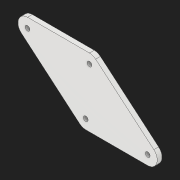
# Autodesk Inventor part: HA014
Saved by Autodesk Inventor 2017 SP1 (Build 210196100, 196)
## iProperties
Created: 2018-02-28
Part Number: HA014
Material: ABS Plastic
Document SubType Name: Modeling
Designer: Zach
Density: 1.06 g/cm^3
Appearance: CR White
Author: Zach
Autodesk Inventor part; units mm, degrees
ref_plane "YZ Plane" through (0, 0, 0) normal (1, 0, 0) x (0, 1, 0)
ref_plane "XZ Plane" through (0, 0, 0) normal (0, 1, 0) x (-1, 0, 0)
ref_plane "XY Plane" through (0, 0, 0) normal (0, 0, 1) x (1, 0, 0)
sketch "Sketch1" plane through (0, 0, 0) normal (0, 0, 1) x (1, 0, 0)
  circle A0 centre (0, 0) radius 2.5
  line L0 (0, 0) -> (65, 0) construction
  line L1 (65, 0) -> (3.9243, 51.6697) construction
  line L2 (0, 0) -> (-61.0757, 51.6697) construction
  line L3 (-61.0757, 51.6697) -> (3.9243, 51.6697) construction
  circle A1 centre (-61.0757, 51.6697) radius 2.5
  circle A2 centre (3.9243, 51.6697) radius 2.5
  circle A3 centre (65, 0) radius 2.5
  line L4 (-88.3791, 61.6697) -> (-3.6625, -10)
  line L5 (-3.6625, -10) -> (92.3034, -10)
  line L6 (92.3034, -10) -> (7.5868, 61.6697)
  line L7 (7.5868, 61.6697) -> (-88.3791, 61.6697)
  dimension "d0" = 5
  dimension "d1" = 65
  dimension "d2" = 80
  dimension "d3" = 5
  dimension "d4" = 5
  dimension "d5" = 5
  dimension "d6" = 139.769
  dimension "d7" = 10
  constraints: 16 end point, 4 centre point, 4 coincident, 4 parallel, 1 horizontal, 3 other
  measures "d0" diameter of A0
  measures "d1" distance of L0.start L0.end
  measures "d2" distance of L0.end L1.end
  measures "d3" diameter of A1
  measures "d4" diameter of A2
  measures "d5" diameter of A3
  measures "d6" angle of L0 L2
  measures "d7" distance between parallel lines of L2 L4
extrude "Extrusion1" add sketch "Sketch1" along normal blind 5
fillet "Fillet1" radius 10 4 edges at (-88.3791, 61.6697, 2.5) (7.5868, 61.6697, 2.5) (92.3034, -10, 2.5) (-3.6625, -10, 2.5)
body "Solid1"
